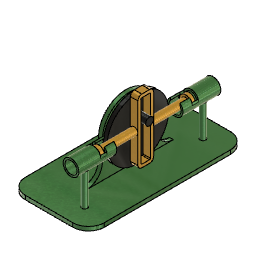
Scotch Yoke v6 (Autodesk Fusion 360 design; units mm, degrees)
Autodesk Fusion 360 part; units mm, degrees
note: some values were not read from the file. Chosen so that the rebuilt part matches the saved one: which face or edge a step refers to. Set by a fixed rule: which sketch regions a step uses.
sketch "support" plane through (0, 0, 0) normal (0, 0, 1) x (1, 0, 0) in component "support"
  line L0 (30, 100) -> (-30, 100)
  line L1 (-50, 80) -> (-50, -80)
  line L2 (-30, -100) -> (30, -100)
  line L3 (50, -80) -> (50, 80)
  arc A0 (-50, -80) -> (-30, -100) centre (-30, -80) ccw
  arc A1 (-30, 100) -> (-50, 80) centre (-30, 80) ccw
  arc A2 (50, 80) -> (30, 100) centre (30, 80) ccw
  arc A3 (30, -100) -> (50, -80) centre (30, -80) ccw
  line L4 (2.5, 40) -> (-2.5, 40)
  line L5 (-2.5, 40) -> (-2.5, -40)
  line L6 (-2.5, -40) -> (2.5, -40)
  line L7 (2.5, -40) -> (2.5, 40)
  point P0 (-50, 100)
  point P1 (-50, -100)
  point P2 (50, -100)
  dimension "d1" = 100
  dimension "d2" = 200
  dimension "d3" = 20
  dimension "d4" = 5
  dimension "d5" = 80
  constraint horizontal L0
  constraint perpendicular L0 L1
  constraint parallel L0 L2
  constraint parallel L1 L3
  constraint coincident P1 L1
  constraint coincident P1 L2
  constraint tangent L1 A0
  constraint tangent L2 A0
  constraint coincident P0 L0
  constraint coincident P0 L1
  constraint tangent L0 A1
  constraint tangent L1 A1
  constraint equal A0 A1
  constraint tangent L0 A2
  constraint tangent L3 A2
  constraint equal A0 A2
  constraint coincident P2 L2
  constraint coincident P2 L3
  constraint tangent L2 A3
  constraint tangent L3 A3
  constraint equal A0 A3
  constraint horizontal L4
  constraint perpendicular L4 L5
  constraint parallel L4 L6
  constraint parallel L5 L7
  measures "d1" distance of P1 P2
  measures "d2" distance of P0 P1
  measures "d3" radius of A0
  measures "d4" distance of L5.end L6.end
  measures "d5" distance of L4.end L5.end
sketch "support legs" plane through (0, 0, 0) normal (0, 0, 1) x (1, 0, 0) in component "support"
  circle A0 centre (30, -80) radius 7.5
  circle A1 centre (30, 80) radius 7.5
  circle A2 centre (-30, -80) radius 7.5
  circle A3 centre (-30, 80) radius 7.5
  point P0 (30, -80)
  point P1 (30, 80)
  point P2 (-30, -80)
  point P3 (-30, 80)
  dimension "d6" = 15
  dimension "d7" = 15
  dimension "d8" = 15
  dimension "d9" = 15
  constraint coincident P0 A0.centre
  constraint coincident P1 A1.centre
  constraint coincident P2 A2.centre
  constraint coincident P3 A3.centre
  measures "d6" diameter of A0
  measures "d7" diameter of A1
  measures "d8" diameter of A2
  measures "d9" diameter of A3
extrude "Extrude1" add sketch "support" along normal blind 5 makes body 1 in component "support"
extrude "Extrude2" add sketch "support" along normal blind 90 contours L4 L5 L6 L7 bodies 1 in component "support"
extrude "Extrude3" add sketch "support legs" against normal blind 7 bodies 1 in component "support"
fillet "Fillet1" radius 20 2 edges at (0, -40, 5) (0, 40, 5) on bodies 1 in component "support"
fillet "Fillet2" radius 40 2 edges at (0, 40, 90) (0, -40, 90) on bodies 1 in component "support"
move_face "OffsetFaces1" offset -5 5 faces at (-0.8333, -40, 33.336) (-0.8333, -1.9109, 89.9547) (0.8333, -0.0027, 90) (0.8333, 39.9547, 51.9109) (0.8333, 40, 33.336) on bodies 1 in component "support"
sketch "support pin" plane through (2.5, 0, 0) normal (1, 0, 0) x (0, 1, 0) in component "support"
  line L0 (-55, 5) -> (55, 5)
  arc A0 (35, 25) -> (55, 5) centre (55, 25) ccw
  line L1 (35, 25) -> (35, 50)
  arc A1 (35, 50) -> (-35, 50) centre (0, 50) ccw
  line L2 (-35, 50) -> (-35, 25)
  arc A2 (-55, 5) -> (-35, 25) centre (-55, 25) ccw
  circle A3 centre (0, 50) radius 5
  circle A4 centre (0, 50) radius 3
  dimension "d21" = 10
  dimension "d22" = -2
  constraint concentric A1 A3
  measures "d21" diameter of A3
extrude "Extrude4" add sketch "support pin" along normal blind 10 contours A4 bodies 1 in component "support"
extrude "Extrude5" add sketch "support pin" along normal blind 5 contours A3 bodies 1 in component "support"
sketch "wheel" plane through (7.5, 0, 0) normal (1, 0, 0) x (0, 1, 0) in component "wheel"
  circle A0 centre (0, 50) radius 3
  circle A1 centre (0, 50) radius 5
  circle A2 centre (0, 50) radius 40
  circle A3 centre (0, 50) radius 3.1
  circle A4 centre (0, 65) radius 5
  dimension "d27" = 80
  dimension "d28" = 6.2
  dimension "d31" = 10
  constraint concentric A0 A2
  constraint concentric A2 A3
  measures "d27" diameter of A2
  measures "d28" diameter of A3
  measures "d31" diameter of A4
extrude "Extrude1'" add sketch "wheel" along normal blind 5 separate body contours A1 | A2 | A4 makes body 2 in component "wheel"
extrude "Extrude2'" add sketch "wheel" along normal blind 15 contours A4 bodies 2 in component "wheel"
sketch "slotted link" plane through (12.5, 0, 0) normal (1, 0, 0) x (0, 1, 0) in component "slotted link"
  circle A0 centre (0, 65) radius 5
  circle A1 centre (0, 50) radius 3.1
  circle A2 centre (0, 50) radius 40
  line L0 (-5, 95) -> (5, 95)
  line L1 (10, 90) -> (10, 19)
  line L2 (5, 14) -> (-5, 14)
  line L3 (-10, 19) -> (-10, 90)
  arc A3 (-5, 95) -> (-10, 90) centre (-5, 90) ccw
  arc A4 (10, 90) -> (5, 95) centre (5, 90) ccw
  arc A5 (-10, 19) -> (-5, 14) centre (-5, 19) ccw
  arc A6 (5, 14) -> (10, 19) centre (5, 19) ccw
  arc A7 (6, 90) -> (5, 91) centre (5, 90) ccw
  line L4 (-5, 91) -> (5, 91)
  arc A8 (-5, 91) -> (-6, 90) centre (-5, 90) ccw
  line L5 (-6, 19) -> (-6, 90)
  arc A9 (-6, 19) -> (-5, 18) centre (-5, 19) ccw
  line L6 (5, 18) -> (-5, 18)
  arc A10 (5, 18) -> (6, 19) centre (5, 19) ccw
  line L7 (6, 90) -> (6, 19)
  point P0 (10, 14)
  point P1 (-10, 14)
  point P2 (0, 50)
  dimension "d34" = 20
  dimension "d35" = 5
  dimension "d36" = 4
  constraint horizontal L0
  constraint perpendicular L0 L1
  constraint parallel L0 L2
  constraint parallel L1 L3
  constraint coincident A1.centre A2.centre
  constraint tangent L0 A3
  constraint tangent L3 A3
  constraint tangent L0 A4
  constraint tangent L1 A4
  constraint equal A3 A4
  constraint coincident P1 L2
  constraint coincident P1 L3
  constraint tangent L2 A5
  constraint tangent L3 A5
  constraint equal A3 A5
  constraint coincident P0 L1
  constraint coincident P0 L2
  constraint tangent L1 A6
  constraint tangent L2 A6
  constraint equal A3 A6
  measures "d34" distance of P0 P1
  measures "d35" radius of A3
extrude "Extrude1''" add sketch "slotted link" along normal blind 10 separate body contours A2 L1 L2 L3 A5 A6 L5 A9 L6 A10 L7 | A2 L0 L1 L3 A3 A4 A7 L4 A8 L5 L7 makes body 3 in component "slotted link"
move_face "OffsetFaces1'" offset -0.5 1 faces at (12.5, -7.3333, 65.7591) on bodies 3 in component "slotted link"
sketch "slotted link right arm" plane through (0, 10, 0) normal (0, 1, 0) x (-1, 0, 0) in component "slotted link"
  line L0 (-13, 19) -> (-13, 90)
  line L1 (-13, 90) -> (-22.5, 90)
  line L2 (-22.5, 90) -> (-22.5, 19)
  line L3 (-22.5, 19) -> (-13, 19)
  line L4 (-22.5, 54.5) -> (-13, 54.5)
  circle A0 centre (-17.75, 54.5) radius 4.75
  dimension "d40" = 9.5
  constraint midpoint L2 L4.start
  constraint midpoint L0 L4.end
  constraint midpoint L4 A0.centre
  measures "d40" diameter of A0
extrude "Extrude2''" add sketch "slotted link right arm" along normal blind 40 contours L4 A0 | L4 A0 bodies 3 in component "slotted link"
sketch "slotted link left arm" plane through (0, -10, 0) normal (0, -1, 0) x (1, 0, 0) in component "slotted link"
  line L0 (13, 90) -> (13, 19)
  line L1 (13, 19) -> (22.5, 19)
  line L2 (22.5, 19) -> (22.5, 90)
  line L3 (22.5, 90) -> (13, 90)
  line L4 (22.5, 54.5) -> (13, 54.5)
  circle A0 centre (17.75, 54.5) radius 4.75
  dimension "d43" = 9.5
  constraint midpoint L2 L4.start
  constraint midpoint L0 L4.end
  constraint midpoint L4 A0.centre
  measures "d43" diameter of A0
extrude "Extrude3'" add sketch "slotted link left arm" along normal blind 40 contours L4 A0 | L4 A0 bodies 3 in component "slotted link"
sketch "right piston head" plane through (0, 50, 0) normal (0, 1, 0) x (-1, 0, 0) in component "slotted link"
  circle A0 centre (-17.75, 54.5) radius 4.75
  circle A1 centre (-17.75, 54.5) radius 7.5
  dimension "d47" = 15
  constraint concentric A0 A1
  measures "d47" diameter of A1
extrude "Extrude4'" add sketch "right piston head" along normal blind 10 contours A0 | A1 bodies 3 in component "slotted link"
sketch "left piston head" plane through (0, -50, 0) normal (0, -1, 0) x (1, 0, 0) in component "slotted link"
  circle A0 centre (17.75, 54.5) radius 4.75
  circle A1 centre (17.75, 54.5) radius 7.5
  dimension "d50" = 15
  constraint concentric A0 A1
  measures "d50" diameter of A1
extrude "Extrude5'" add sketch "left piston head" along normal blind 10 contours A0 | A1 bodies 3 in component "slotted link"
sketch "right piston tube" plane through (0, 60, 0) normal (0, 1, 0) x (-1, 0, 0) in component "support"
  circle A0 centre (-17.75, 54.5) radius 7.5
  circle A1 centre (-17.75, 54.5) radius 10
  circle A2 centre (-17.75, 54.5) radius 7.7
  dimension "d57" = 20
  dimension "d58" = -2.3
  constraint concentric A0 A1
  measures "d57" diameter of A1
extrude "Extrude6" add sketch "right piston tube" along normal blind 40 and the other way blind 10 separate body contours A1 makes body 4 in component "support"
sketch "left piston tube" plane through (0, -60, 0) normal (0, -1, 0) x (1, 0, 0) in component "support"
  circle A0 centre (17.75, 54.5) radius 7.5
  circle A1 centre (17.75, 54.5) radius 10
  circle A2 centre (17.75, 54.5) radius 7.7
  dimension "d63" = 20
  dimension "d64" = -2.3
  constraint concentric A0 A1
  measures "d63" diameter of A1
extrude "Extrude7" add sketch "left piston tube" along normal blind 40 and the other way blind 15 separate body contours A1 makes body 5 in component "support"
extrude "Extrude8" add 1 faces at (8.5539, 50, 54.0032) along direction (0, -1, 0) blind 5 on bodies 4 bodies 4 in component "support"
sketch "piston tubes legs" plane through (0, 0, 5) normal (0, 0, 1) x (-1, 0, 0) in component "support"
  arc A0 (-30, 100) -> (-50, 80) centre (-30, 80) ccw
  line L0 (-50, 80) -> (-50, -80)
  arc A1 (-50, -80) -> (-30, -100) centre (-30, -80) ccw
  line L1 (-30, -100) -> (30, -100)
  arc A2 (30, -100) -> (50, -80) centre (30, -80) ccw
  line L2 (50, -80) -> (50, 80)
  arc A3 (50, 80) -> (30, 100) centre (30, 80) ccw
  line L3 (30, 100) -> (-30, 100)
  line L4 (-2.5, -55) -> (-2.5, 55)
  line L5 (-2.5, 55) -> (2.5, 55)
  line L6 (2.5, 55) -> (2.5, -55)
  line L7 (2.5, -55) -> (-2.5, -55)
  circle A4 centre (-20, 75) radius 7.5
  circle A5 centre (-20, -75) radius 3.5
  dimension "d71" = 15
  measures "d71" diameter of A4
extrude "Extrude9" add sketch "piston tubes legs" along normal blind 41 contours A4 | A5 bodies 1 in component "support"
move_face "OffsetFaces2" offset -4 1 faces at (12.5093, -74.6262, 32.3333) on bodies 1 in component "support"
combine "Combine1" operation add target body 1 tool bodies 4 5 in component "support"
move_face "OffsetFaces1''" offset -0.05 1 faces at (15.8333, 4.9752, 65.4978) on bodies 2 in component "wheel"
move_face "OffsetFaces2'" offset -5 1 faces at (11.2123, 50, 53.8914) on bodies 3 in component "slotted link"
move_face "OffsetFaces3" offset -5 1 faces at (24.3054, -50, 54.8726) on bodies 3 in component "slotted link"
move_face "OffsetFaces3'" offset -1 1 faces at (9.1667, 39.9503, 51.9938) on bodies 2 in component "wheel"
extrude "Extrude3''" add 1 faces at (22.5, 1.3817, 66.1754) along direction (1, 0, 0) blind 5 on bodies 2 bodies 2 in component "wheel"
ref_plane "WorkPlane2" through (18, -51, 55) normal (0, 0, 1) x (-1, 0, 0) in component "support"
sketch "left piston holder cut" plane through (18, -51, 55) normal (0, 0, 1) x (1, 0, 0) in component "support"
  line L0 (-6, 11) -> (6, 11)
  line L1 (6, 11) -> (6, -3)
  line L2 (6, -3) -> (9, -3)
  line L3 (9, -3) -> (9, -11)
  line L4 (9, -11) -> (-9, -11)
  line L5 (-9, -11) -> (-9, -3)
  line L6 (-9, -3) -> (-6, -3)
  line L7 (-6, -3) -> (-6, 11)
  constraint horizontal L0
  constraint perpendicular L0 L1
  constraint perpendicular L1 L2
  constraint perpendicular L2 L3
  constraint perpendicular L3 L4
  constraint perpendicular L4 L5
  constraint perpendicular L5 L6
  constraint perpendicular L0 L7
extrude "Extrude10" cut sketch "left piston holder cut" along normal blind 20 bodies 1 in component "support"
ref_plane "WorkPlane3" through (18, 51, 55) normal (0, 0, 1) x (-1, 0, 0) in component "support"
sketch "right piston holder cut" plane through (18, 51, 55) normal (0, 0, 1) x (1, 0, 0) in component "support"
  line L0 (-9, 11) -> (-9, 3)
  line L1 (-9, 3) -> (-6, 3)
  line L2 (-6, 3) -> (-6, -11)
  line L3 (-6, -11) -> (6, -11)
  line L4 (6, -11) -> (6, 3)
  line L5 (6, 3) -> (9, 3)
  line L6 (9, 3) -> (9, 11)
  line L7 (9, 11) -> (-9, 11)
  constraint vertical L0
  constraint perpendicular L0 L1
  constraint perpendicular L1 L2
  constraint perpendicular L2 L3
  constraint perpendicular L3 L4
  constraint perpendicular L4 L5
  constraint perpendicular L5 L6
  constraint perpendicular L0 L7
extrude "Extrude11" cut sketch "right piston holder cut" along normal blind 20 bodies 1 in component "support"
move_face "OffsetFaces3''" offset 3 1 faces at (26.3295, -45, 57.8622) on bodies 1 in component "support"
move_face "OffsetFaces4" offset 3 1 faces at (24.0091, 45, 47.7372) on bodies 1 in component "support"
move_face "OffsetFaces5" offset -10 1 faces at (26.9461, -100, 54.0032) on bodies 1 in component "support"
move_face "OffsetFaces6" offset -10 1 faces at (8.5539, 100, 54.0032) on bodies 1 in component "support"
component "Scotch Yoke" placed x (1, 0, 0) y (0, 1, 0) z (0, 0, 1) at (0, 0, 0)
component "support" placed x (1, 0, 0) y (0, 1, 0) z (0, 0, 1) at (0, 0, 0) in component "Scotch Yoke"
component "wheel" placed x (1, 0, 0) y (0, 1, 0) z (0, 0, 1) at (0, 0, 0) in component "support"
component "slotted link" placed x (1, 0, 0) y (0, 1, 0) z (0, 0, 1) at (0, 0, 0) in component "wheel"
named bodies: "support", "right piston tube", "left piston tube"
